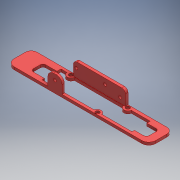
# Autodesk Inventor part: xtion_custom_heatsink_mount
Saved by Autodesk Inventor 2017 (Build 210142000, 142)
## iProperties
Created: 2016-11-28
Part Number: xtion_custom_heatsink_mount
Material: PC/ABS Plastic
Document SubType Name: Modeling
Designer: Alistair
Density: 0.357273 g/cm^3
Appearance: Smooth - Red
Author: Alistair
## iProperties of the stored document xtion_custom_heatsink_mount_3DPrint.ipt
Created: 2016-11-28
Part Number: xtion_custom_heatsink_mount_3DPrint
Material: Generic
Document SubType Name: Modeling
Designer: Alistair
Density: 1 g/cm^3
Appearance: Default
Author: Alistair
Autodesk Inventor part; units mm, degrees
ref_plane "YZ Plane" through (0, 0, 0) normal (1, 0, 0) x (0, 1, 0)
ref_plane "XZ Plane" through (0, 0, 0) normal (0, 1, 0) x (-1, 0, 0)
ref_plane "XY Plane" through (0, 0, 0) normal (0, 0, 1) x (1, 0, 0)
sketch "Sketch1" plane through (0, 0, 0) normal (0, 0, 1) x (1, 0, 0)
  circle A0 centre (29.8658, 2.0543) radius 1.1 construction
  circle A1 centre (-34.1342, 2.0543) radius 1.1 construction
  circle A2 centre (17.3658, -19.4457) radius 1.1 construction
  arc A3 (77.5658, -1.4457) -> (71.0658, 5.0543) centre (71.0658, -1.4457) ccw construction
  line L0 (-75.3342, 5.0543) -> (71.0658, 5.0543) construction
  arc A4 (-75.3342, 5.0543) -> (-81.8342, -1.4457) centre (-75.3342, -1.4457) ccw construction
  line L1 (-81.8342, -3.2457) -> (-81.8342, -1.4457) construction
  arc A5 (-81.8342, -3.2457) -> (-77.5665, -5.0135) centre (-79.3342, -3.2457) ccw construction
  line L2 (-75.4025, -2.8495) -> (-77.5665, -5.0135) construction
  arc A6 (-70.8063, -0.9457) -> (-75.4025, -2.8495) centre (-70.8063, -7.4457) ccw construction
  line L3 (7.8658, -0.9457) -> (-70.8063, -0.9457) construction
  arc A7 (14.3658, -7.4457) -> (7.8658, -0.9457) centre (7.8658, -7.4457) ccw construction
  line L4 (14.3658, -14.9457) -> (14.3658, -7.4457) construction
  line L5 (14.3658, -21.9457) -> (14.3658, -14.9457) construction
  line L6 (20.3658, -21.9457) -> (14.3658, -21.9457) construction
  line L7 (20.3658, -14.9457) -> (20.3658, -21.9457) construction
  line L8 (20.3658, -7.4457) -> (20.3658, -14.9457) construction
  arc A8 (26.8658, -0.9457) -> (20.3658, -7.4457) centre (26.8658, -7.4457) ccw construction
  line L9 (67.2302, -0.9457) -> (26.8658, -0.9457) construction
  arc A9 (69.7302, -1.4457) -> (67.2302, -0.9457) centre (67.2302, -7.4457) ccw construction
  line L10 (73.298, -5.0135) -> (69.7302, -1.4457) construction
  arc A10 (73.298, -5.0135) -> (77.5658, -3.2457) centre (75.0658, -3.2457) ccw construction
  line L11 (77.5658, -1.4457) -> (77.5658, -3.2457) construction
  circle A11 centre (17.3658, -15.6457) radius 0.75 construction
  circle A12 centre (-79.3342, -3.2457) radius 0.75 construction
  circle A13 centre (75.0658, -3.2457) radius 0.75 construction
  circle A14 centre (17.3658, -3.2457) radius 0.75 construction
  line L12 (-75.3342, 5.0543) -> (71.0658, 5.0543)
  line L13 (77.5658, -1.4457) -> (77.5658, -21.9457)
  line L14 (77.5658, -21.9457) -> (-81.8342, -21.9457)
  line L15 (-81.8342, -21.9457) -> (-81.8342, -1.4457)
  arc A15 (-75.3342, 5.0543) -> (-81.8342, -1.4457) centre (-75.3342, -1.4457) ccw projected
  arc A16 (77.5658, -1.4457) -> (71.0658, 5.0543) centre (71.0658, -1.4457) ccw projected
  point P0 (0, 0)
  constraints: 8 end point, 4 point on circle, 2 parallel, 1 horizontal, 1 perpendicular
extrude "Extrusion1" add sketch "Sketch1" along normal blind 3
sketch "Sketch2" plane through (0, 0, 3) normal (0, 0, 1) x (1, 0, 0)
  circle A0 centre (29.8658, 2.0543) radius 1.1 projected
  circle A1 centre (-34.1342, 2.0543) radius 1.1 projected
  circle A2 centre (17.3658, -19.4457) radius 1.1 projected
  point P0 (0, 0)
hole "Hole1" at (-34.1342, 2.0543, 3) at (17.3658, -19.4457, 3) at (29.8658, 2.0543, 3) direction (0, 0, -1) diameter 2.3 end through all counterbore diameter 4.5 counterbore depth 2.2
sketch "Sketch3" plane through (0, 0, 3) normal (0, 0, 1) x (1, 0, 0)
  line L0 (69.2331, -2.2265) -> (69.2331, -16.2835)
  line L1 (-61.3045, -16.2835) -> (-61.3045, -2.2265)
  circle A0 centre (-34.1342, 2.0543) radius 2.25 construction
  circle A1 centre (-34.1342, 2.0543) radius 1.15 construction
  circle A2 centre (29.8658, 2.0543) radius 2.25 construction
  circle A3 centre (29.8658, 2.0543) radius 1.15 construction
  circle A4 centre (17.3658, -19.4457) radius 2.25 construction
  circle A5 centre (17.3658, -19.4457) radius 1.15 construction
  arc A6 (-38.6902, 2.2735) -> (-29.7413, 1.5975) centre (-34.1902, 2.2735) ccw
  line L2 (-45.5022, 2.2735) -> (-38.6902, 2.2735)
  line L3 (-29.7413, 1.5975) -> (25.4168, 1.5975)
  line L4 (34.3147, 1.5975) -> (55.7139, 1.5975)
  arc A7 (25.4168, 1.5975) -> (34.3147, 1.5975) centre (29.8658, 2.2735) ccw
  line L5 (55.7139, -19.0025) -> (21.7425, -19.0025)
  line L6 (12.989, -19.0025) -> (-45.5022, -19.0025)
  arc A8 (21.7425, -19.0025) -> (12.989, -19.0025) centre (17.3658, -20.0483) ccw
  line L7 (-53.8342, -3.5957) -> (-53.8342, -15.2957) projected
  line L8 (-56.8342, -15.2957) -> (-56.8342, -3.5957) projected
  line L9 (-53.8342, -15.2957) -> (-56.8342, -15.2957) projected
  line L10 (-56.8342, -3.5957) -> (-53.8342, -3.5957) projected
  line L11 (63.8658, -15.5457) -> (63.8658, -3.3457) projected
  line L12 (66.6658, -3.3457) -> (66.6658, -15.5457) projected
  line L13 (66.6658, -15.5457) -> (63.8658, -15.5457) projected
  line L14 (63.8658, -3.3457) -> (66.6658, -3.3457) projected
  line L15 (-45.5022, 2.2735) -> (-45.5022, -2.2265)
  line L16 (-45.5022, -2.2265) -> (-61.3045, -2.2265)
  line L17 (-45.5022, -16.2835) -> (-45.5022, -19.0025)
  line L18 (-45.5022, -16.2835) -> (-61.3045, -16.2835)
  line L19 (55.7139, 1.5975) -> (55.7139, -2.2265)
  line L20 (55.7139, -2.2265) -> (69.2331, -2.2265)
  line L21 (55.7139, -19.0025) -> (55.7139, -16.2835)
  line L22 (55.7139, -16.2835) -> (69.2331, -16.2835)
  point P0 (0, 0)
  dimension "d9" = 4.5
  dimension "d10" = 4.5
  dimension "d11" = 4.5
  dimension "d15" = 20.6
  constraints: 30 end point, 7 parallel, 7 perpendicular, 6 point on circle, 4 collinear, 4 point on line, 3 centre point, 3 horizontal, 2 vertical
  measures "d9" radius of A6
  measures "d10" radius of A7
  measures "d11" radius of A8
  measures "d15" distance between parallel lines of L6 L3
extrude "Extrusion2" cut sketch "Sketch3" against normal through all contours L0 L22 L21 L5 A8 L6 L17 L18 L1 L16 L15 L2 A6 L3 A7 L4 L19 L20 | L7 L9 L8 L10 | L11 L14 L12 L13
fillet "Fillet1" radius 7.75 2 edges at (-81.8342, -21.9457, 1.5) (77.5658, -21.9457, 1.5)
sketch "Sketch4" plane through (-75.3342, 5.0543, 0) normal (0, 1, 0) x (1, 0, 0)
  line L0 (44.0825, -3) -> (102.5284, -3)
  line L1 (102.5284, -3) -> (102.5284, -19)
  line L2 (102.5284, -19) -> (44.0825, -19)
  line L3 (44.0825, -19) -> (44.0825, -3)
  line L4 (146.4, -3) -> (0, -3) projected
  point P0 (75.3342, 0)
  dimension "d16" = 16
  constraints: 8 end point, 2 parallel, 1 collinear, 1 horizontal, 1 perpendicular
  measures "d16" distance between parallel lines of L2 L0
extrude "Extrusion3" add sketch "Sketch4" against normal blind 3
sketch "Sketch5" plane through (-74.0842, -21.9457, 0) normal (0, -1, 0) x (1, 0, 0)
  line L0 (143.9, 3) -> (143.9, 0) projected
  line L1 (0, 3) -> (143.9, 3) projected
  line L2 (0, 0) -> (0, 3) projected
  line L3 (0, 0) -> (143.9, 0) projected
  line L4 (0, 3) -> (143.9, 3) projected
  line L5 (101.2784, 19) -> (42.8325, 19) projected
  line L6 (38.0287, 3) -> (54.0287, 3)
  line L7 (54.0287, 3) -> (54.0287, 19)
  line L8 (54.0287, 19) -> (38.0287, 19)
  line L9 (38.0287, 19) -> (38.0287, 3)
  point P0 (74.0842, 0)
  point P1 (89.4899, 23)
  point P2 (57.4899, 23)
  dimension "d25" = 16
  constraints: 8 end point, 2 parallel, 1 horizontal, 1 perpendicular, 1 point on line, 2 other
  measures "d25" distance between parallel lines of L7 L9
extrude "Extrusion4" add sketch "Sketch5" against normal blind 2.5 contours L1 L9 L8 L5 L7
fillet "Fillet3" radius 4 2 edges at (-31.2517, 3.5543, 19) (27.1942, 3.5543, 19)
fillet "Fillet4" radius 3.25 4 edges at (-61.3045, -2.2265, 1.5) (-61.3045, -16.2835, 1.5) (69.2331, -2.2265, 1.5) (69.2331, -16.2835, 1.5)
fillet "Fillet5" radius 6.5 2 edges at (-36.0555, -20.6957, 19) (-20.0555, -20.6957, 19)
sketch "Sketch7" plane through (-74.0842, -21.9457, 0) normal (0, -1, 0) x (1, 0, 0)
  point P0 (74.0842, 0)
  point P1 (46.0287, 12.8596)
  point P2 (95.4084, 8.91)
  point P3 (78.425, 12.9132)
hole "Hole2" at (-28.0555, -21.9457, 12.8596) at (21.3241, -21.9457, 8.91) at (4.3407, -21.9457, 12.9132) direction (0, 1, 0) diameter 3.2 end through all
body "Solid1"
